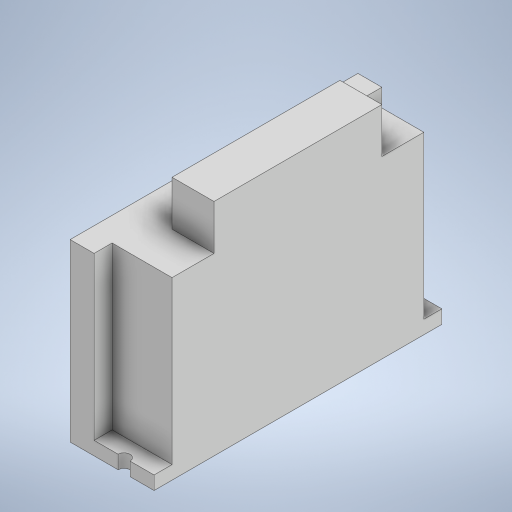
# Autodesk Inventor part: driver
Saved by Autodesk Inventor 2024 (Build 280153000, 153)
## iProperties
Created: 2024-04-22
Part Number: driver
Material: Generic
Document SubType Name: Modeling
Designer: MaartenGeorgesBuelen
Density: 1 g/cm^3
Appearance: Default
Author: MaartenGeorgesBuelen
Autodesk Inventor part; units mm, degrees
ref_plane "YZ Plane" through (0, 0, 0) normal (1, 0, 0) x (0, 1, 0)
ref_plane "XZ Plane" through (0, 0, 0) normal (0, 1, 0) x (-1, 0, 0)
ref_plane "XY Plane" through (0, 0, 0) normal (0, 0, 1) x (1, 0, 0)
sketch "Sketch3" plane through (0, 0, 0) normal (0, 1, 0) x (-1, 0, 0)
  line L0 (0, 0) -> (28, 0)
  line L1 (28, 0) -> (28, -96)
  line L2 (28, -96) -> (0, -96)
  line L3 (0, -96) -> (0, 0)
  dimension "d6" = 28
  dimension "d7" = 96
  constraints: 8 end point, 2 parallel, 1 horizontal, 1 perpendicular
  measures "d6" distance of L1.end L2.end
  measures "d7" distance of L0.end L1.end
extrude "Extrusion3" add sketch "Sketch3" along normal blind 4.5
sketch "Sketch4" plane through (0, 4.5, 0) normal (0, 1, 0) x (1, 0, 0)
  line L0 (0, 96) -> (-28, 96) projected
  line L1 (-28, 96) -> (-28, 0) projected
  line L2 (-28, 0) -> (0, 0) projected
  line L3 (0, 0) -> (0, 96) projected
  line L4 (-28, 0) -> (-20, 0)
  line L5 (-20, 0) -> (-20, 96)
  line L6 (-20, 96) -> (-28, 96)
  line L7 (-28, 96) -> (-28, 0)
  line L8 (0, 0) -> (-20, 0)
  line L9 (-20, 0) -> (-20, 6)
  line L10 (-20, 6) -> (0, 6)
  line L11 (0, 6) -> (0, 0)
  line L12 (0, 96) -> (-20, 96)
  line L13 (-20, 96) -> (-20, 90)
  line L14 (-20, 90) -> (0, 90)
  line L15 (0, 90) -> (0, 96)
  dimension "d10" = 8
  dimension "d11" = 6
  dimension "d12" = 6
  constraints: 24 end point, 6 parallel, 3 horizontal, 3 perpendicular, 3 point on line
  measures "d10" distance of L6.end L5.end
  measures "d11" distance of L8.end L9.end
  measures "d12" distance of L13.end L12.end
extrude "Extrusion4" add sketch "Sketch4" along normal blind 54 contours L5 L2 L1 L0 | L3 L10 L5 L14
sketch "Sketch5" plane through (0, 4.5, 0) normal (0, 1, 0) x (1, 0, 0)
  line L0 (0, 6) -> (-20, 6) projected
  line L1 (-20, 6) -> (-20, 0) projected
  line L2 (-20, 0) -> (0, 0) projected
  line L3 (0, 0) -> (0, 6) projected
  circle A0 centre (-10, 0) radius 2
  line L4 (-20, 96) -> (-20, 90) projected
  line L5 (-20, 90) -> (0, 90) projected
  line L6 (0, 90) -> (0, 96) projected
  line L7 (0, 96) -> (-20, 96) projected
  circle A1 centre (-10, 96) radius 2
  point P0 (-8, 0)
  point P1 (-12, 0)
  dimension "d15" = 4
  dimension "d16" = 4
  constraints: 2 centre point, 2 midpoint
  measures "d15" diameter of A0
  measures "d16" diameter of A1
extrude "Extrusion5" cut sketch "Sketch5" against normal through all contours L2 A0 | A1 L7 | L7 A1 picked at (-9.3527, 0.1595)
sketch "Sketch6" plane through (0, 58.5, 0) normal (0, 1, 0) x (1, 0, 0)
  line L0 (-20, 6) -> (0, 6) projected
  line L1 (0, 6) -> (0, 90) projected
  line L2 (0, 90) -> (-20, 90) projected
  line L3 (-20, 90) -> (-20, 96) projected
  line L4 (-20, 96) -> (-28, 96) projected
  line L5 (-28, 96) -> (-28, 0) projected
  line L6 (-28, 0) -> (-20, 0) projected
  line L7 (-20, 0) -> (-20, 6) projected
  line L8 (0, 20) -> (-14, 20)
  line L9 (-14, 20) -> (-14, 76)
  line L10 (-14, 76) -> (0, 76)
  line L11 (0, 76) -> (0, 20)
  point P0 (0, 0)
  point P1 (0, 76)
  dimension "d19" = 14
  dimension "d21" = 14
  dimension "d22" = 14
  constraints: 8 end point, 2 parallel, 1 horizontal, 1 perpendicular, 1 point on line
  measures "d19" distance between parallel lines of L0 L8
  measures "d21" distance between parallel lines of L2 L10
  measures "d22" distance between parallel lines of L1 L9
extrude "Extrusion6" add sketch "Sketch6" along normal blind 15 contours L8 L9 L10 L1
body "Solid2"
